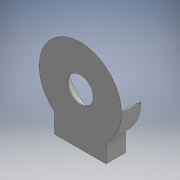
# Autodesk Inventor part: cup
Saved by Autodesk Inventor 2016 (Build 200138000, 138)
## iProperties
Created: 2016-05-03
Part Number: cup
Material: Generic
Document SubType Name: Modeling
Designer: mkepler
Density: 1 g/cm^3
Appearance: Default
Author: mkepler
Autodesk Inventor part; units mm, degrees
ref_plane "YZ Plane" through (0, 0, 0) normal (1, 0, 0) x (0, 1, 0)
ref_plane "XZ Plane" through (0, 0, 0) normal (0, 1, 0) x (-1, 0, 0)
ref_plane "XY Plane" through (0, 0, 0) normal (0, 0, 1) x (1, 0, 0)
sketch "Sketch1" plane through (0, 0, 0) normal (0, 0, 1) x (1, 0, 0)
  line L0 (0, 0) -> (20.5, 0)
  line L1 (20.5, 0) -> (20.5, 2)
  line L2 (20.5, 0) -> (25.5, 0)
  line L3 (25.5, 0) -> (20.5, 2)
  line L4 (0, 0) -> (0, 3)
  dimension "d0" = 20.5
  dimension "d1" = 2
  dimension "d2" = 5
  constraints: 10 end point, 2 horizontal, 1 perpendicular, 1 vertical
  measures "d0" distance of L0.start L0.end
  measures "d1" distance of L0.end L1.end
  measures "d2" distance of L0.end L2.end
revolve "Revolution1" add sketch "Sketch1" angle 360 about axis through (0, 0, 0) along (0, 1, 0)
sketch "Sketch2" plane through (0, 0, 0) normal (0, -1, 0) x (1, 0, 0)
  circle A0 centre (0, 0) radius 22
  constraints: 1 centre point, 1 coincident
extrude "Extrusion1" add sketch "Sketch2" against normal blind 0.5
sketch "Sketch3" plane through (0, 0.5, 0) normal (0, 1, 0) x (1, 0, 0)
  circle A0 centre (0, 0) radius 8
  dimension "d6" = 16
  constraints: 1 centre point, 1 coincident
  measures "d6" diameter of A0
extrude "Extrusion2" cut sketch "Sketch3" against normal blind 0.5
sketch "Sketch4" plane through (0, 0, 0) normal (0, -1, 0) x (1, 0, 0)
  circle A0 centre (0, 0) radius 25.5 projected
  line L0 (-15.9375, -26.9259) -> (-15.9375, -19.9059)
  line L1 (15.9375, -26.9259) -> (15.9375, -19.9059)
  circle A1 centre (0, 0) radius 8 projected
  arc A2 (-15.9375, -19.9059) -> (15.9375, -19.9059) centre (0, 0) ccw
  line L2 (15.9375, -26.9259) -> (15.9375, -31.9259)
  line L3 (15.9375, -31.9259) -> (-15.9375, -31.9259)
  line L4 (-15.9375, -31.9259) -> (-15.9375, -26.9259)
  constraints: 10 end point, 4 point on circle, 1 centre point, 1 coincident, 1 collinear, 1 concentric, 1 perpendicular, 1 vertical
extrude "Extrusion3" add sketch "Sketch4" against normal blind 3 contours A0 L1 L2 L3 L4 L0
sketch "Sketch10" plane through (0, 3, 0) normal (0, 1, 0) x (1, 0, 0)
  arc A0 (25.5, -0.0165) -> (-25.5, -0.047) centre (0, 0) ccw
  arc A1 (19.9722, 4.6218) -> (-19.9809, 4.584) centre (0, 0) ccw
  arc A2 (-15.9375, 19.9059) -> (15.9375, 19.9059) centre (0, 0) ccw projected
  line L0 (-25.5, -0.047) -> (-19.9809, 4.584)
  circle A3 centre (0, 0) radius 20.5 projected
  line L1 (-25.5, -0.047) -> (-18.2954, -0.047) construction
  line L2 (25.5, -0.0165) -> (19.9722, 4.6218)
  dimension "d33" = 40
  constraints: 8 point on circle, 6 end point, 2 centre point, 2 coincident, 1 equal length, 1 horizontal
  measures "d33" angle of L1 L0
extrude "Extrusion7" add sketch "Sketch10" against normal through all contours L2 A1 L0 A0
sketch "Sketch11" plane through (0, 3, 0) normal (0, 1, 0) x (1, 0, 0)
  arc A0 (19.9722, 4.6218) -> (-19.9809, 4.584) centre (0, 0) ccw
  arc A1 (25.5, -0.0165) -> (15.9375, 19.9059) centre (0, 0) ccw projected
  line L0 (15.9375, 31.9259) -> (15.9375, 19.9059) projected
  line L1 (15.9375, 19.9059) -> (15.9375, 31.9259)
  line L2 (-15.9375, 31.9259) -> (15.9375, 31.9259) projected
  line L3 (15.9375, 31.9259) -> (-15.9375, 31.9259)
  arc A2 (-15.9375, 19.9059) -> (-25.5, -0.047) centre (0, 0) ccw projected
  line L4 (-15.9375, 31.9259) -> (-15.9375, 19.9059)
  line L5 (19.9722, 4.6218) -> (25.5, -0.0165) projected
  line L6 (19.9722, 4.6218) -> (25.5, -0.0165)
  line L7 (-25.5, -0.047) -> (-19.9809, 4.584) projected
  line L8 (-25.5, -0.047) -> (-19.9809, 4.584)
  arc A3 (-15.9375, 19.9059) -> (-25.5, -0.047) centre (0, 0) ccw
  arc A4 (25.5, -0.0165) -> (15.9375, 19.9059) centre (0, 0) ccw
  constraints: 10 end point, 6 point on circle, 4 collinear, 3 centre point, 2 coincident, 1 perpendicular
extrude "Extrusion8" add sketch "Sketch11" along normal blind 9
sketch "Sketch12" plane through (15.9375, 0, -31.9259) normal (0, 0, -1) x (-1, 0, 0)
  line L0 (15.9375, 0) -> (15.9375, 12)
  line L1 (0, 12) -> (31.875, 12) projected
  circle A0 centre (21.9375, 6.5) radius 2.175
  line L2 (31.875, 0) -> (0, 0) projected
  circle A1 centre (9.9375, 6.5) radius 2.175
  dimension "d39" = 4.35
  dimension "d40" = 6.5
  dimension "d41" = 4.35
  dimension "d42" = 6
  dimension "d43" = 6
  dimension "d51" = 6.5
  constraints: 2 centre point, 2 end point, 1 midpoint
  measures "d39" diameter of A0
  measures "d40" distance from line of L2 A0.centre
  measures "d41" diameter of A1
  measures "d42" distance from line of L0 A1.centre
  measures "d43" distance from line of L0 A0.centre
  measures "d51" distance from line of L2 A1.centre
hole "Hole2" at (6, 6.5, -31.9259) at (-6, 6.5, -31.9259) direction (0, 0, 1) diameter 4.35 depth 8 tip angle 118
body "Solid1"
